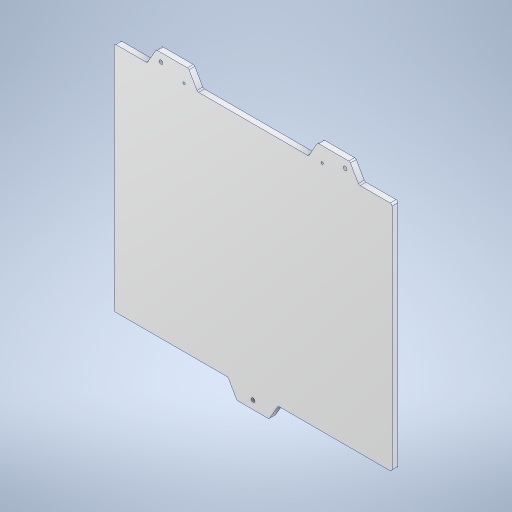
# Autodesk Inventor part: Print Bed
Saved by Autodesk Inventor 2024 (Build 280153000, 153)
## iProperties
Created: 2024-08-02
Part Number: Print Bed
Material: Aluminum 6061
Document SubType Name: Modeling
Designer: Ishaan
Density: 2.7 g/cm^3
Appearance: Aluminum - Flat
Author: Ishaan
Autodesk Inventor part; units mm, degrees
ref_plane "YZ Plane" through (0, 0, 0) normal (1, 0, 0) x (0, 1, 0)
ref_plane "XZ Plane" through (0, 0, 0) normal (0, 1, 0) x (-1, 0, 0)
ref_plane "XY Plane" through (0, 0, 0) normal (0, 0, 1) x (1, 0, 0)
sketch "Sketch1" plane through (0, 0, 0) normal (0, 0, 1) x (1, 0, 0)
  line L0 (151, -126) -> (-151, -126)
  line L1 (-151, -126) -> (-151, 126)
  line L2 (-151, 126) -> (151, 126)
  line L3 (151, 126) -> (151, -126)
  line L4 (151, -126) -> (-151, 126) construction
  line L5 (-151, -126) -> (151, 126) construction
  point P0 (0, 0)
  dimension "d0" = 302
  dimension "d1" = 252
  constraints: 12 end point, 2 midpoint, 2 parallel, 1 horizontal, 1 perpendicular
  measures "d0" distance of L1.end L2.end
  measures "d1" distance of L0.end L1.end
extrude "Extrusion1" add sketch "Sketch1" along normal blind 6.35
sketch "Sketch2" plane through (0, 0, 6.35) normal (0, 0, 1) x (1, 0, 0)
  line L0 (-110.3923, 134) -> (-105.1962, 143)
  line L1 (-105.1962, 143) -> (-94.8038, 143)
  line L2 (-94.8038, 143) -> (-89.6077, 134)
  line L3 (-89.6077, 134) -> (-94.8038, 125)
  line L4 (-94.8038, 125) -> (-105.1962, 125)
  line L5 (-105.1962, 125) -> (-110.3923, 134)
  line L6 (94.8038, 143) -> (105.1962, 143)
  line L7 (105.1962, 143) -> (110.3923, 134)
  line L8 (110.3923, 134) -> (105.1962, 125)
  line L9 (105.1962, 125) -> (94.8038, 125)
  line L10 (94.8038, 125) -> (89.6077, 134)
  line L11 (89.6077, 134) -> (94.8038, 143)
  line L12 (-100, 134) -> (100, 134) construction
  line L13 (151, 126) -> (-151, 126) projected
  line L14 (-105.1962, 143) -> (-115.0111, 126)
  line L15 (105.1962, 143) -> (115.0111, 126)
  line L16 (94.8038, 143) -> (-94.8038, 143)
  line L17 (-151, -126) -> (151, -126) projected
  line L18 (-27.315, -126) -> (-17.5, -143)
  line L19 (-17.5, -143) -> (17.5, -143)
  line L20 (17.5, -143) -> (27.315, -126)
  line L21 (-70.1962, 143) -> (-60.3812, 126)
  line L22 (60.3812, 126) -> (70.1962, 143)
  point P0 (0, 0)
  point P1 (0, 134)
  point P2 (0, -143)
  point P3 (0, -134)
  dimension "d4" = 18
  dimension "d5" = 200
  dimension "d6" = 8
  dimension "d7" = 17
  dimension "d8" = 17
  dimension "d9" = 35
  dimension "d10" = 8
  dimension "d32" = 35
  dimension "d33" = 35
  constraints: 42 end point, 8 point on line, 5 parallel, 4 collinear, 3 vertical alignment, 2 coincident, 2 horizontal, 2 midpoint, 26 other
  measures "d4" distance between parallel lines of L4 L1
  measures "d5" distance of L12.start L12.end
  measures "d6" distance between parallel lines of L13 L12
  measures "d7" distance between parallel lines of L19 L17
  measures "d8" distance between parallel lines of L13 L16
  measures "d9" distance of L18.end L19.end
  measures "d10" distance from line of L17 point (0, -134)
  measures "d32" distance of L21.start L0.end
  measures "d33" distance of L6.end L22.end
extrude "Extrusion2" add sketch "Sketch2" against normal up to surface (6.35 mm away) contours L0 L1 L2 L3 L13 L5 | L5 L13 L14 | L16 L21 L13 L3 L2 | L16 L11 L10 L13 L22 | L6 L7 L8 L13 L10 L11 | L8 L15 L13 | L17 L20 L19 L18
hole "Hole1" at (0, -134, 6.35) at (-100, 134, 6.35) at (100, 134, 6.35) direction (0, 0, -1) diameter 4.134 end through all thread size "M5x0.8" class "6H" standard "ANSI Metric M Profile"
fillet "Fillet1" radius 2 16 edges at (17.5, -143, 3.175) (27.315, -126, 3.175) (151, -126, 3.175) (-151, 126, 3.175) (115.0111, 126, 3.175) (105.1962, 143, 3.175) (151, 126, 3.175) (-27.315, -126, 3.175) (-17.5, -143, 3.175) (-151, -126, 3.175) (-115.0111, 126, 3.175) (-105.1962, 143, 3.175) (-70.1962, 143, 3.175) (-60.3812, 126, 3.175) (60.3812, 126, 3.175) (70.1962, 143, 3.175)
sketch "Sketch3" plane through (0, 0, 6.35) normal (0, 0, 1) x (1, 0, 0)
  line L0 (150, -125) -> (-150, -125) construction
  line L1 (-150, -125) -> (-150, 125) construction
  line L2 (-150, 125) -> (150, 125) construction
  line L3 (150, 125) -> (150, -125) construction
  line L4 (150, -125) -> (-150, 125) construction
  line L5 (-150, -125) -> (150, 125) construction
  circle A0 centre (-75, 126.6) radius 1.6 construction
  line L6 (-75, 126.6) -> (75, 126.6) construction
  circle A1 centre (75, 126.6) radius 1.6 construction
  point P0 (0, 0)
  point P1 (0, 126.6)
  dimension "d21" = 300
  dimension "d22" = 250
  dimension "d23" = 3.2
  dimension "d24" = 150
  constraints: 14 end point, 3 coincident, 3 midpoint, 2 centre point, 2 horizontal, 2 parallel, 1 equal radius, 1 perpendicular, 1 tangent, 1 vertical alignment
  measures "d21" distance of L1.end L2.end
  measures "d22" distance of L0.end L1.end
  measures "d23" diameter of A0
  measures "d24" distance of L6.start L6.end
hole "Hole2" at (-75, 126.6, 6.35) at (75, 126.6, 6.35) direction (0, 0, -1) diameter 2.459 end through all thread size "M3x0.5" class "6H" standard "ANSI Metric M Profile"
equation "\"d7\" = d8"
equation "\"d10\" = d6"
equation "\"d32\" = d9"
equation "\"d33\" = d32"
body "Solid1"
